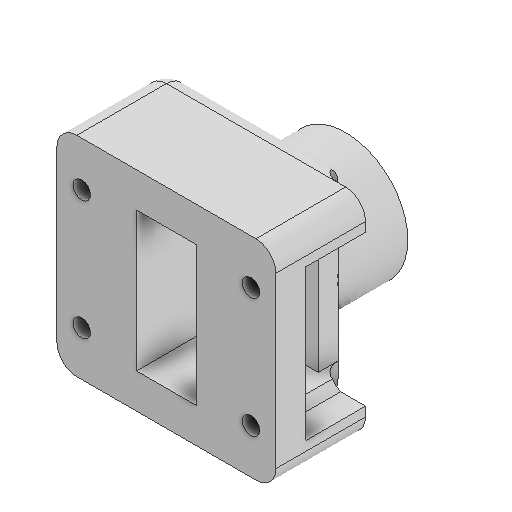
# Autodesk Inventor part: 210312 - Mirrorcle MEMS mount for half inch v4
Saved by Autodesk Inventor 2022 (Build 260153000, 153)
## iProperties
Created: 2021-03-12
Part Number: 210312 - Mirrorcle MEMS mount for half inch v4
Material: Generic
Document SubType Name: Modeling
Designer: Ralf
Density: 1 g/cm^3
Appearance: Default
Author: Ralf
Autodesk Inventor part; units mm, degrees
ref_plane "YZ Plane" through (0, 0, 0) normal (1, 0, 0) x (0, 1, 0)
ref_plane "XZ Plane" through (0, 0, 0) normal (0, 1, 0) x (-1, 0, 0)
ref_plane "XY Plane" through (0, 0, 0) normal (0, 0, 1) x (1, 0, 0)
sketch "Sketch1" plane through (0, 0, 0) normal (0, 0, 1) x (1, 0, 0)
  line L0 (-11, 10.5) -> (11, 10.5)
  line L1 (11, 10.5) -> (11, -10.5)
  line L2 (11, -10.5) -> (-11, -10.5)
  line L3 (-11, -10.5) -> (-11, 10.5)
  line L4 (-3, 7) -> (3, 7)
  line L5 (3, 7) -> (3, -7)
  line L6 (3, -7) -> (-3, -7)
  line L7 (-3, -7) -> (-3, 7)
  point P0 (0, 0)
  dimension "d0" = 22
  dimension "d1" = 21
  dimension "d2" = 10.5
  dimension "d3" = 11
  dimension "d6" = 6
  dimension "d7" = 3
  dimension "d8" = 14
  dimension "d9" = 7
  constraints: 16 end point, 4 parallel, 2 horizontal, 2 perpendicular
  measures "d0" distance of L0.start L0.end
  measures "d1" distance of L2.end L0.start
  measures "d2" distance from line of point (0, 0) L2
  measures "d3" distance from line of point (0, 0) L3
  measures "d6" distance of L4.start L4.end
  measures "d7" distance from line of point (0, 0) L7
  measures "d8" distance between parallel lines of L6 L4
  measures "d9" distance from line of point (0, 0) L6
extrude "Extrusion1" add sketch "Sketch1" along normal blind 4
sketch "Sketch2" plane through (0, 0, 0) normal (0, 0, -1) x (-1, 0, 0)
  circle A0 centre (8.5, -6) radius 0.875
  circle A1 centre (8.5, 6) radius 0.875
  circle A2 centre (-8.5, -6) radius 0.875
  circle A3 centre (-8.5, 6) radius 0.875
  point P0 (0, 0)
  dimension "d10" = 1.75
  dimension "d11" = 1.75
  dimension "d12" = 1.75
  dimension "d13" = 1.75
  dimension "d14" = 6
  dimension "d15" = 6
  dimension "d16" = 8.5
  dimension "d17" = 8.5
  dimension "d18" = 8.5
  dimension "d19" = 6
  dimension "d20" = 6
  dimension "d21" = 8.5
  constraints: 4 centre point
  measures "d10" diameter of A0
  measures "d11" diameter of A1
  measures "d12" diameter of A2
  measures "d13" diameter of A3
  measures "d14" vertical distance of point (0, 0) A0.centre
  measures "d15" vertical distance of A1.centre point (0, 0)
  measures "d16" horizontal distance of point (0, 0) A1.centre
  measures "d17" horizontal distance of point (0, 0) A0.centre
  measures "d18" horizontal distance of point (0, 0) A2.centre
  measures "d19" vertical distance of point (0, 0) A2.centre
  measures "d20" vertical distance of point (0, 0) A3.centre
  measures "d21" horizontal distance of point (0, 0) A3.centre
extrude "Extrusion2" cut sketch "Sketch2" against normal blind 4
sketch "Sketch3" plane through (0, 0, 0) normal (0, 0, -1) x (-1, 0, 0)
  circle A0 centre (8.5, -6) radius 0.875 projected
  line L0 (9.85, -6.7794) -> (8.5, -7.5588)
  line L1 (8.5, -7.5588) -> (7.15, -6.7794)
  line L2 (7.15, -6.7794) -> (7.15, -5.2206)
  line L3 (7.15, -5.2206) -> (8.5, -4.4412)
  line L4 (8.5, -4.4412) -> (9.85, -5.2206)
  line L5 (9.85, -5.2206) -> (9.85, -6.7794)
  circle A1 centre (8.5, 6) radius 0.875 projected
  line L6 (9.85, 5.2206) -> (8.5, 4.4412)
  line L7 (8.5, 4.4412) -> (7.15, 5.2206)
  line L8 (7.15, 5.2206) -> (7.15, 6.7794)
  line L9 (7.15, 6.7794) -> (8.5, 7.5588)
  line L10 (8.5, 7.5588) -> (9.85, 6.7794)
  line L11 (9.85, 6.7794) -> (9.85, 5.2206)
  circle A2 centre (-8.5, -6) radius 0.875 projected
  line L12 (-9.85, -5.2206) -> (-8.5, -4.4412)
  line L13 (-8.5, -4.4412) -> (-7.15, -5.2206)
  line L14 (-7.15, -5.2206) -> (-7.15, -6.7794)
  line L15 (-7.15, -6.7794) -> (-8.5, -7.5588)
  line L16 (-8.5, -7.5588) -> (-9.85, -6.7794)
  line L17 (-9.85, -6.7794) -> (-9.85, -5.2206)
  circle A3 centre (-8.5, 6) radius 0.875 projected
  line L18 (-9.85, 6.7794) -> (-8.5, 7.5588)
  line L19 (-8.5, 7.5588) -> (-7.15, 6.7794)
  line L20 (-7.15, 6.7794) -> (-7.15, 5.2206)
  line L21 (-7.15, 5.2206) -> (-8.5, 4.4412)
  line L22 (-8.5, 4.4412) -> (-9.85, 5.2206)
  line L23 (-9.85, 5.2206) -> (-9.85, 6.7794)
  line L24 (11, 10.5) -> (11, -10.5) projected
  line L25 (11, -4.1525) -> (11, -7.963)
  line L26 (11, 7.8475) -> (11, 4.037)
  line L27 (-11, -10.5) -> (-11, 10.5) projected
  line L28 (-11, -4.1525) -> (-11, -7.963)
  line L29 (-11, 7.8475) -> (-11, 4.037)
  line L30 (-11, -10.5) -> (-11, 10.5) projected
  line L31 (-11, 7.5588) -> (-11, 4.1525)
  line L32 (11, 7.5588) -> (11, 3.8638)
  line L33 (11, 10.5) -> (11, -10.5) projected
  line L34 (11, -4.4412) -> (11, -8.1362)
  line L35 (-11, -4.4412) -> (-11, -7.963)
  line L36 (-8.5, 7.5588) -> (-11, 7.5588)
  line L37 (-11, 7.5588) -> (-11, 4.4412)
  line L38 (-11, 4.4412) -> (-8.5, 4.4412)
  line L39 (-8.5, 4.4412) -> (-8.5, 7.5588)
  line L40 (-8.5, -4.4412) -> (-11, -4.4412)
  line L41 (-11, -4.4412) -> (-11, -7.5588)
  line L42 (-11, -7.5588) -> (-8.5, -7.5588)
  line L43 (-8.5, -7.5588) -> (-8.5, -4.4412)
  line L44 (8.5, -4.4412) -> (11, -4.4412)
  line L45 (11, -4.4412) -> (11, -7.5588)
  line L46 (11, -7.5588) -> (8.5, -7.5588)
  line L47 (8.5, -7.5588) -> (8.5, -4.4412)
  line L48 (8.5, 7.5588) -> (11, 7.5588)
  line L49 (11, 7.5588) -> (11, 4.4412)
  line L50 (11, 4.4412) -> (8.5, 4.4412)
  line L51 (8.5, 4.4412) -> (8.5, 7.5588)
  point P0 (0, 0)
  dimension "d24" = 2.7
  dimension "d25" = 2.7
  dimension "d26" = 2.7
  dimension "d27" = 2.7
  constraints: 96 end point, 10 point on line, 8 parallel, 4 coincident, 4 horizontal, 4 perpendicular, 55 other
  measures "d24" distance between parallel lines of L2 L5
  measures "d25" distance between parallel lines of L8 L11
  measures "d26" distance between parallel lines of L17 L14
  measures "d27" distance between parallel lines of L20 L23
extrude "Extrusion3" cut sketch "Sketch3" against normal blind 1.8 contours A0 L47 | A0 L47 L4 L5 L0 | L47 A0 | A0 L47 L1 L2 L3 | L44 L24 L46 L0 L5 L4 | A1 L51 | A1 L51 L10 L11 L6 | L51 A1 | A1 L51 L7 L8 L9 | L48 L24 L50 L6 L11 L10 | A2 L43 | A2 L43 L13 L14 L15 | L43 A2 | A2 L43 L16 L17 L12 | L12 L17 L16 L42 L27 L40 | A3 L39 L19 L20 L21 | A3 L39 L22 L23 L18 | L18 L23 L22 L38 L27 L36
sketch "Sketch4" plane through (0, 0, 0) normal (0, 0, -1) x (-1, 0, 0)
  line L0 (11, 10.5) -> (11, -10.5) projected
  line L1 (11, -10.5) -> (-11, -10.5) projected
  line L2 (11, 10.5) -> (3, 10.5)
  line L3 (3, 10.5) -> (3, -10.5)
  line L4 (3, -10.5) -> (11, -10.5)
  line L5 (11, -10.5) -> (11, 10.5)
  line L6 (-11, -7.5588) -> (-11, -4.4412) projected
  line L7 (3, -10.5) -> (-11, -10.5)
  line L8 (-11, -10.5) -> (-11, -7)
  line L9 (-11, -7) -> (3, -7)
  line L10 (3, -7) -> (3, -10.5)
  line L11 (3, 10.5) -> (-11, 10.5)
  line L12 (-11, 10.5) -> (-11, 7)
  line L13 (-11, 7) -> (3, 7)
  line L14 (3, 7) -> (3, 10.5)
  circle A0 centre (-8.5, 6) radius 0.875 projected
  line L15 (-7.15, 6.7794) -> (-7.15, 5.2206) projected
  line L16 (-7.15, 5.2206) -> (-8.5, 4.4412)
  line L17 (-8.5, 4.4412) -> (-9.85, 5.2206)
  line L18 (-9.85, 5.2206) -> (-9.85, 6.7794)
  line L19 (-9.85, 6.7794) -> (-8.5, 7.5588)
  line L20 (-8.5, 7.5588) -> (-7.15, 6.7794)
  line L21 (-7.15, 6.7794) -> (-7.15, 5.2206)
  line L22 (-7.15, -6.7794) -> (-8.5, -7.5588)
  line L23 (-8.5, -7.5588) -> (-9.85, -6.7794)
  line L24 (-9.85, -6.7794) -> (-9.85, -5.2206)
  line L25 (-9.85, -5.2206) -> (-8.5, -4.4412)
  line L26 (-8.5, -4.4412) -> (-7.15, -5.2206)
  line L27 (-7.15, -5.2206) -> (-7.15, -6.7794)
  line L28 (-11, 7.5588) -> (-8.5, 7.5588) projected
  line L29 (-8.5, 7.5588) -> (-11, 7.5588)
  line L30 (-11, 7.5588) -> (-11, 7)
  line L31 (-9.4679, 7) -> (-8.5, 7.5588)
  line L32 (-7.15, -6.7794) -> (-8.5, -7.5588) projected
  line L33 (-8.5, -7.5588) -> (-11, -7.5588) projected
  line L34 (-8.5, -7.5588) -> (-11, -7.5588)
  line L35 (-11, -7.5588) -> (-11, -7)
  line L36 (-9.4679, -7) -> (-8.5, -7.5588)
  point P0 (0, 0)
  point P1 (11, 7.8475)
  point P2 (-11, -7.963)
  point P3 (-11, -4.1525)
  point P4 (-7.15, 6)
  point P5 (-8.5, -6)
  point P6 (-7.15, -6)
  point P7 (-7.5321, 7)
  point P8 (-7.5321, -7)
  dimension "d30" = 8
  dimension "d31" = 3.5
  dimension "d32" = 14
  dimension "d33" = 3.5
  constraints: 60 end point, 7 point on line, 6 parallel, 4 horizontal, 4 perpendicular, 3 collinear, 3 midpoint, 1 coincident, 26 other
  measures "d30" distance of L4.end L3.end
  measures "d31" distance of L7.end L8.end
  measures "d32" distance of L13.end L12.end
  measures "d33" distance of L12.end L11.end
extrude "Extrusion4" add sketch "Sketch4" along normal blind 6 contours L0 L1 L3 L2 | L3 L13 L20 L28 L12 L11 | L1 L8 L33 L22 L9 L3
sketch "Sketch5" plane through (0, 0, -6) normal (0, 0, -1) x (-1, 0, 0)
  circle A0 centre (0, 0) radius 6.25
  line L0 (11, -10.5) -> (11, 10.5) projected
  line L1 (11, -10.5) -> (-11, -10.5) projected
  line L2 (11, 10.5) -> (-6.25, 10.5)
  line L3 (-6.25, 10.5) -> (-6.25, -10.5)
  line L4 (-6.25, -10.5) -> (11, -10.5)
  line L5 (11, -10.5) -> (11, 10.5)
  dimension "d36" = 12.5
  constraints: 8 end point, 2 parallel, 1 centre point, 1 coincident, 1 horizontal, 1 perpendicular, 1 point on line
  measures "d36" diameter of A0
extrude "Extrusion5" add sketch "Sketch5" along normal blind 2 contours A0 | L3 L2 L0 L1
sketch "Sketch6" plane through (0, 0, -8) normal (0, 0, -1) x (-1, 0, 0)
  circle A0 centre (0, 0) radius 6.25
  dimension "d39" = 12.5
  constraints: 1 centre point, 1 coincident
  measures "d39" diameter of A0
extrude "Extrusion6" add sketch "Sketch6" along normal blind 7
sketch "Sketch7" plane through (0, 0, 4) normal (0, 0, 1) x (1, 0, 0)
  line L0 (-11, 10.5) -> (-11, -10.5) projected
  line L1 (11, -10.5) -> (11, 10.5) projected
  line L2 (-11, 10.5) -> (11, 10.5)
  line L3 (11, 10.5) -> (11, -10.5)
  line L4 (11, -10.5) -> (-11, -10.5)
  line L5 (-11, -10.5) -> (-11, 10.5)
  point P0 (0, 0)
  constraints: 8 end point, 2 parallel, 1 horizontal, 1 perpendicular
extrude "Extrusion7" cut sketch "Sketch7" against normal blind 1
fillet "Fillet1" radius 2 9 edges at (11, 10.5, -1.5) (-11, 10.5, -2.5) (11, -10.5, -1.5) (-11, -10.5, -2.5) (6.25, 8.75, -6) (6.25, -8.75, -6) (-2.375, -10.5, -8) (-11, 0, -8) (-2.375, 10.5, -8)
sketch "Sketch9" plane through (0, 0, 0) normal (0, 0, 1) x (1, 0, 0)
  line L0 (-8.5, 7.5588) -> (-11, 7.5588) projected
  line L1 (-11, 7.5588) -> (-8.5, 7.5588)
  line L2 (-8.5, 7.5588) -> (-8.5, 4.4412)
  line L3 (-8.5, 4.4412) -> (-11, 4.4412)
  line L4 (-11, 4.4412) -> (-11, 7.5588)
  line L5 (-8.5, 7.5588) -> (-7.15, 6.7794)
  line L6 (-7.15, 5.2206) -> (-7.15, 6.7794) projected
  line L7 (-7.15, 6.7794) -> (-7.15, 5.2206)
  line L8 (-7.15, 5.2206) -> (-8.5, 4.4412)
  line L9 (-8.5, 4.4412) -> (-8.5, 7.5588)
  line L10 (-8.5, -4.4412) -> (-11, -4.4412) projected
  line L11 (-11, -4.4412) -> (-8.5, -4.4412)
  line L12 (-8.5, -4.4412) -> (-8.5, -7.5588)
  line L13 (-8.5, -7.5588) -> (-11, -7.5588)
  line L14 (-11, -7.5588) -> (-11, -4.4412)
  line L15 (-8.5, -4.4412) -> (-7.15, -5.2206)
  line L16 (-7.15, -5.2206) -> (-7.218, -6.7794)
  line L17 (-7.218, -6.7794) -> (-8.5, -7.5588)
  point P0 (0, 0)
  constraints: 30 end point, 6 equal length, 2 horizontal, 2 perpendicular
extrude "Extrusion9" cut sketch "Sketch9" against normal blind 20
sketch "Sketch10" plane through (0, 0, 1.8) normal (0, 0, -1) x (-1, 0, 0)
  circle A0 centre (8.5, -6) radius 0.875 projected
  line L0 (7.15, -6.7794) -> (7.15, -5.2206) projected
  line L1 (7.15, -5.2206) -> (8.5, -4.4412)
  line L2 (8.5, -4.4412) -> (9.85, -5.2206)
  line L3 (9.85, -5.2206) -> (9.85, -6.7794)
  line L4 (9.85, -6.7794) -> (8.5, -7.5588)
  line L5 (8.5, -7.5588) -> (7.15, -6.7794)
  line L6 (7.15, -6.7794) -> (7.15, -5.2206)
  circle A1 centre (8.5, 6) radius 0.875 projected
  line L7 (7.15, 5.2206) -> (7.15, 6.7794) projected
  line L8 (7.15, 6.7794) -> (8.5, 7.5588)
  line L9 (8.5, 7.5588) -> (9.85, 6.7794)
  line L10 (9.85, 6.7794) -> (9.85, 5.2206)
  line L11 (9.85, 5.2206) -> (8.5, 4.4412)
  line L12 (8.5, 4.4412) -> (7.15, 5.2206)
  line L13 (7.15, 5.2206) -> (7.15, 6.7794)
  line L14 (11, -7.5588) -> (8.5, -7.5588) projected
  line L15 (11, -7.5588) -> (8.5, -7.5588)
  line L16 (8.5, -7.5588) -> (8.5, -4.4412)
  line L17 (8.5, -4.4412) -> (11, -4.4412)
  line L18 (11, -4.4412) -> (11, -7.5588)
  line L19 (11, -4.4412) -> (11, 4.4412) projected
  line L20 (11, 4.4412) -> (8.5, 4.4412)
  line L21 (8.5, 4.4412) -> (8.5, 7.5588)
  line L22 (8.5, 7.5588) -> (11, 7.5588)
  line L23 (11, 7.5588) -> (11, 4.4412)
  circle A2 centre (-8.5, 6) radius 0.875 projected
  line L24 (-7.15, 6.7794) -> (-7.15, 5.2206) projected
  line L25 (-7.15, 5.2206) -> (-8.5, 4.4412)
  line L26 (-8.5, 4.4412) -> (-9.85, 5.2206)
  line L27 (-9.85, 5.2206) -> (-9.85, 6.7794)
  line L28 (-9.85, 6.7794) -> (-8.5, 7.5588)
  line L29 (-8.5, 7.5588) -> (-7.15, 6.7794)
  line L30 (-7.15, 6.7794) -> (-7.15, 5.2206)
  circle A3 centre (-8.5, -6) radius 0.875 projected
  line L31 (-7.15, -5.2206) -> (-7.15, -6.7794) projected
  line L32 (-7.15, -6.7794) -> (-8.5, -7.5588)
  line L33 (-8.5, -7.5588) -> (-9.85, -6.7794)
  line L34 (-9.85, -6.7794) -> (-9.85, -5.2206)
  line L35 (-9.85, -5.2206) -> (-8.5, -4.4412)
  line L36 (-8.5, -4.4412) -> (-7.15, -5.2206)
  line L37 (-7.15, -5.2206) -> (-7.15, -6.7794)
  line L38 (-11, 7.5588) -> (-8.5, 7.5588) projected
  line L39 (-11, 8.5) -> (-11, -8.5) projected
  line L40 (-8.5, 7.5588) -> (-11, 7.5588)
  line L41 (-11, 7.5588) -> (-11, 4.4412)
  line L42 (-11, 4.4412) -> (-8.5, 4.4412)
  line L43 (-8.5, 4.4412) -> (-8.5, 7.5588)
  line L44 (-11, -4.4412) -> (-8.5, -4.4412) projected
  line L45 (-8.5, -4.4412) -> (-11, -4.4412)
  line L46 (-11, -4.4412) -> (-11, -7.5588)
  line L47 (-11, -7.5588) -> (-8.5, -7.5588)
  line L48 (-8.5, -7.5588) -> (-8.5, -4.4412)
  point P0 (0, 0)
  point P1 (7.15, -6)
  point P2 (7.15, 6)
  point P3 (-7.15, 6)
  point P4 (-7.15, -6)
  constraints: 80 end point, 8 midpoint, 8 parallel, 4 coincident, 4 horizontal, 4 perpendicular, 2 point on line, 52 other
extrude "Extrusion10" add sketch "Sketch10" along normal blind 1.8 contours L17 L18 L14 L4 L3 L2 | L22 L23 L20 L11 L10 L9 | L28 L27 L26 L42 L39 L38 | L35 L34 L33 L47 L39 L44
sketch "Sketch12" plane through (0, 0, -8) normal (0, 0, -1) x (-1, 0, 0)
  circle A0 centre (8.5, -6) radius 0.875 projected
  circle A1 centre (8.5, -6) radius 2
  circle A2 centre (8.5, 6) radius 0.875 projected
  circle A3 centre (8.5, 6) radius 2
  point P0 (0, 0)
  dimension "d51" = 4
  dimension "d52" = 4
  constraints: 2 centre point, 2 coincident
  measures "d51" diameter of A1
  measures "d52" diameter of A3
extrude "Extrusion11" cut sketch "Sketch12" against normal blind 8 contours A0 | A1 | A2 | A3
body "Solid1"
